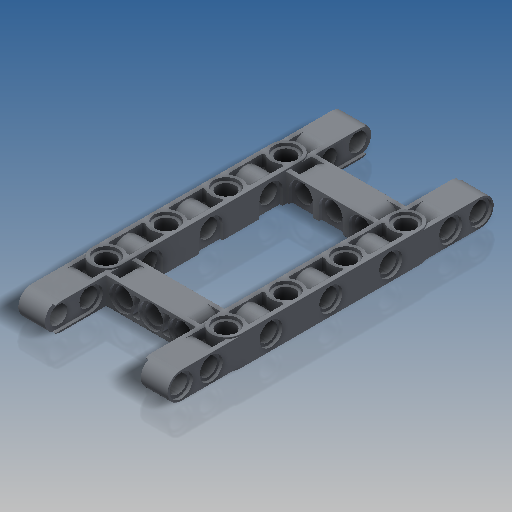
# Autodesk Inventor part: 64178-LtBluishGray
Saved by Autodesk Inventor 2018.3 (Build 223284000, 284)
## iProperties
Created: 2012-03-21
Part Number: 64178-LtBluishGray
Document SubType Name: Modeling
Designer: D. Kohfeld
Density: 1.06 g/cm^3
Material: ABS Plastic
Mass: 7.50717 g
Surface Area: 111.293 cm^2
Volume: 7.08223 cm^3
Appearance: LtBluishGray
Author: D. Kohfeld
Autodesk Inventor part; units mm, degrees
ref_plane "XZ Plane" through (0, 0, 0) normal (0, 1, 0) x (-1, 0, 0)
ref_plane "XY Plane" through (0, 0, 0) normal (0, 0, 1) x (1, 0, 0)
sketch "Sketch1" plane through (0, 0, 0) normal (0, 0, 1) x (1, 0, 0)
  line L0 (4, -24) -> (4, 24)
  line L1 (-4, 24) -> (-4, -24)
  arc A0 (4, 24) -> (-4, 24) centre (0, 24) ccw
  arc A1 (-4, -24) -> (4, -24) centre (0, -24) ccw
  circle A2 centre (0, 24) radius 3.2
  circle A3 centre (0, 24) radius 2.4
  line L2 (2.8284, 21.1716) -> (2.8284, 10.8284)
  line L3 (-2.8284, 21.1716) -> (-2.8284, 10.8284)
  arc A4 (-2.8284, 21.1716) -> (2.8284, 21.1716) centre (0, 24) ccw
  arc A5 (2.8284, 10.8284) -> (-2.8284, 10.8284) centre (0, 8) ccw
  circle A6 centre (0, 8) radius 3.2
  circle A7 centre (0, 8) radius 2.4
  line L4 (2.8284, 5.1716) -> (2.8284, -5.1716)
  line L5 (-2.8284, 5.1716) -> (-2.8284, -5.1716)
  arc A8 (-2.8284, 5.1716) -> (2.8284, 5.1716) centre (0, 8) ccw
  arc A9 (2.8284, -5.1716) -> (-2.8284, -5.1716) centre (0, -8) ccw
  circle A10 centre (0, -8) radius 3.2
  circle A11 centre (0, -8) radius 2.4
  line L6 (2.8284, -10.8284) -> (2.8284, -21.1716)
  line L7 (-2.8284, -10.8284) -> (-2.8284, -21.1716)
  arc A12 (-2.8284, -10.8284) -> (2.8284, -10.8284) centre (0, -8) ccw
  arc A13 (2.8284, -21.1716) -> (-2.8284, -21.1716) centre (0, -24) ccw
  circle A14 centre (0, -24) radius 3.2
  circle A15 centre (0, -24) radius 2.4
  line L8 (-4, -24) -> (-4, -40)
  line L9 (-4, -40) -> (-2.8284, -40)
  line L10 (-2.8284, -40) -> (-2.8284, -26.8284)
  line L11 (4, -24) -> (4, -40)
  line L12 (4, -40) -> (2.8284, -40)
  line L13 (2.8284, -40) -> (2.8284, -26.8284)
  line L14 (-4, 24) -> (-4, 40)
  line L15 (-4, 40) -> (-2.8284, 40)
  line L16 (-2.8284, 40) -> (-2.8284, 26.8284)
  line L17 (4, 24) -> (4, 40)
  line L18 (4, 40) -> (2.8284, 40)
  line L19 (2.8284, 40) -> (2.8284, 26.8284)
  line L20 (-2.8284, -40) -> (2.8284, -40)
  line L21 (-2.8284, 40) -> (2.8284, 40)
  line L22 (-2.8284, 21.1716) -> (0, 24) construction
  point P0 (0, 0)
  point P1 (-4, 0)
  dimension "d32" = 8
  dimension "d49" = 6.4
  dimension "d50" = 4.8
  dimension "d64" = 16
  dimension "d105" = 16
  dimension "d116" = 45
  constraints: 46 end point, 20 point on circle, 16 centre point, 10 parallel, 9 coincident, 8 tangent, 6 vertical alignment, 5 perpendicular, 4 equal radius, 3 equal length, 3 horizontal alignment, 3 vertical, 2 concentric, 1 midpoint, 28 other
  measures "d32" diameter of A0
  measures "d49" diameter of A2
  measures "d50" diameter of A3
  measures "d64" distance of L3.start L5.start
  measures "d105" vertical distance of L11.end A1.centre
  measures "d116" angle of L1 L22
extrude "Extrusion1" add sketch "Sketch1" along normal mid plane 8 contours A1 L1 A0 L0 | A2 | L2 A5 L3 A4 | A6 | L4 A9 L5 A8 | A10 | L6 A13 L7 A12 | A14
extrude "Extrusion18" add sketch "Sketch1" along normal mid plane 7.2 contours L11 L12 L13 A1 | A0 L19 L18 L17 | L10 L9 L8 A1 | A0 L14 L15 L16
sketch "Sketch6" plane through (0, 0, 4) normal (0, 0, 1) x (1, 0, 0)
  circle A0 centre (0, 24) radius 2.4 projected
  circle A1 centre (0, 24) radius 3.2 projected
  line L0 (2.8284, 21.1716) -> (2.8284, 10.8284) projected
  arc A2 (-2.8284, 21.1716) -> (2.8284, 21.1716) centre (0, 24) ccw projected
  arc A3 (2.8284, 10.8284) -> (-2.8284, 10.8284) centre (0, 8) ccw projected
  line L1 (-2.8284, 21.1716) -> (-2.8284, 10.8284) projected
  circle A4 centre (0, 8) radius 3.2 projected
  circle A5 centre (0, 24) radius 3.1 projected
  circle A6 centre (0, 8) radius 3.1 projected
  line L2 (4, 24) -> (4, -24) projected
  line L3 (4, -24) -> (4, 24) projected
  arc A7 (-2.8284, 5.1716) -> (2.8284, 5.1716) centre (0, 8) ccw projected
  line L4 (2.8284, 5.1716) -> (2.8284, -5.1716) projected
  arc A8 (2.8284, -5.1716) -> (-2.8284, -5.1716) centre (0, -8) ccw projected
  line L5 (-2.8284, 5.1716) -> (-2.8284, -5.1716) projected
  circle A9 centre (0, -8) radius 3.2 projected
  line L6 (2.8284, -10.8284) -> (2.8284, -21.1716) projected
  arc A10 (-2.8284, -10.8284) -> (2.8284, -10.8284) centre (0, -8) ccw projected
  line L7 (-2.8284, -10.8284) -> (-2.8284, -21.1716) projected
  arc A11 (2.8284, -21.1716) -> (-2.8284, -21.1716) centre (0, -24) ccw projected
  circle A12 centre (0, -24) radius 3.2 projected
  line L8 (4, -40) -> (4, -24) projected
  line L9 (4, -24) -> (4, -40) projected
  line L10 (4, 40) -> (4, 24) projected
  line L11 (4, 24) -> (4, 40) projected
extrude "Extrusion7" cut sketch "Sketch6" against normal blind 0.8 contours A0 | A1 | A4 | A5 | A6 | A9 | A12
extrude "Extrusion8" cut sketch "Sketch6" against normal blind 3.1 contours L0 A3 L1 A2 | A7 L4 A8 L5 | L6 A11 L7 A10
mirror "Mirror1" about plane through (0, 0, 0) normal (0, 0, 1) of "Extrusion7", "Extrusion8"
extrude "Extrusion19" add sketch "Sketch1" against normal up to surface (1.8 mm away) from surface at 0.9 contours L13 L20 L10 A1 | A0 L16 L21 L19
sketch "Sketch7" plane through (0, 0, 0) normal (1, 0, 0) x (0, 1, 0)
  line L0 (-21.1716, 0.9) -> (-10.8284, 0.9) projected
  line L1 (-21.1716, -0.9) -> (-10.8284, -0.9) projected
  circle A0 centre (-16, 0) radius 3.6
  circle A1 centre (-16, 0) radius 2.4
  circle A2 centre (0, 0) radius 3.6
  circle A3 centre (0, 0) radius 2.4
  circle A4 centre (16, 0) radius 3.6
  circle A5 centre (16, 0) radius 2.4
  line L2 (-16, 0) -> (0, 0) construction
  line L3 (0, 0) -> (16, 0) construction
  line L4 (-40, -3.6) -> (-40, 3.6) construction
  line L5 (40, -3.6) -> (40, 3.6) construction
  arc A6 (-40, 3.6) -> (-40, -3.6) centre (-40, 0) ccw
  arc A7 (40, -3.6) -> (40, 3.6) centre (40, 0) ccw
  line L6 (-40, 3.6) -> (-32, 3.6)
  arc A8 (-32, -3.6) -> (-32, 3.6) centre (-32, 0) ccw
  line L7 (-32, -3.6) -> (-40, -3.6)
  line L8 (40, 3.6) -> (32, 3.6)
  arc A9 (32, 3.6) -> (32, -3.6) centre (32, 0) ccw
  line L9 (32, -3.6) -> (40, -3.6)
  line L10 (-40, 0) -> (-32, 0) construction
  line L11 (32, 0) -> (40, 0) construction
  circle A10 centre (-40, 0) radius 3.2
  circle A11 centre (-32, 0) radius 3.2
  circle A12 centre (-32, 0) radius 2.4
  circle A13 centre (-40, 0) radius 2.4
  circle A14 centre (32, 0) radius 3.2
  circle A15 centre (40, 0) radius 3.2
  circle A16 centre (40, 0) radius 2.4
  circle A17 centre (32, 0) radius 2.4
  point P0 (-16, 0.9)
  dimension "d69" = 7.2
  dimension "d70" = 4.8
  dimension "d108" = 8
  dimension "d109" = 6.4
  dimension "d110" = 4.8
  constraints: 18 centre point, 16 end point, 12 coincident, 10 equal radius, 8 point on circle, 8 tangent, 5 parallel, 4 collinear, 3 midpoint, 1 horizontal alignment, 1 perpendicular, 1 vertical alignment
  measures "d69" diameter of A0
  measures "d70" diameter of A1
  measures "d108" distance of L10.end L10.start
  measures "d109" diameter of A10
  measures "d110" diameter of A13
extrude "Extrusion9" add sketch "Sketch7" against normal up to surface (8 mm away) from surface at 4 contours A0 L0 A1 | L0 A1 L1 A0 | A0 L1 A1 L0 | L1 A1 A0 | A2 | A4 | L6 A8 L7 A6 | L9 A9 L8 A7 | A10 | A11 | A14 | A15
extrude "Extrusion10" cut sketch "Sketch7" along normal through all both and the other way through all contours A1 L0 | L0 A1 L1 | L1 A1 | A3 | A5 | A12 | A13 | A16 | A17
sketch "Sketch8" plane through (4, -24, 4) normal (1, 0, 0) x (0, 0, -1)
  circle A0 centre (4, 24) radius 2.4 projected
  circle A1 centre (4, 8) radius 2.4 projected
  circle A2 centre (4, 40) radius 2.4 projected
  circle A3 centre (4, 8) radius 3.1
  circle A4 centre (4, 24) radius 3.1
  circle A5 centre (4, 40) radius 3.1
  circle A6 centre (4, 56) radius 2.4 projected
  circle A7 centre (4, -8) radius 2.4 projected
  arc A8 (0.4, -16) -> (7.6, -16) centre (4, -16) ccw projected
  arc A9 (7.6, 64) -> (0.4, 64) centre (4, 64) ccw projected
  circle A10 centre (4, 56) radius 3.1
  circle A11 centre (4, 64) radius 3.1
  circle A12 centre (4, -8) radius 3.1
  circle A13 centre (4, -16) radius 3.1
  dimension "d75" = 6.2
  constraints: 7 centre point, 7 coincident, 6 equal radius
  measures "d75" diameter of A3
extrude "Extrusion11" cut sketch "Sketch8" against normal blind 0.8
mirror "Mirror2" about plane through (0, 0, 0) normal (1, 0, 0) of "Extrusion11"
sketch "Sketch18" plane through (-4, -24, -4) normal (-1, 0, 0) x (0, 0, 1)
  circle A0 centre (4, 40) radius 3.1 projected
  circle A1 centre (4, 8) radius 3.1 projected
  circle A2 centre (4, 24) radius 3.1 projected
  line L0 (0, 48) -> (0, 0) projected
  line L1 (4, 43.1) -> (0, 43.1)
  line L2 (4, 36.9) -> (0, 36.9)
  line L3 (4, 27.1) -> (0, 27.1)
  line L4 (4, 20.9) -> (0, 20.9)
  line L5 (4, 11.1) -> (0, 11.1)
  line L6 (4, 4.9) -> (0, 4.9)
  constraints: 12 end point, 6 perpendicular, 6 point on circle, 6 point on line, 6 tangent
extrude "Extrusion26" cut sketch "Sketch18" against normal up to surface (0.8 mm away) contours A0 L2 L0 L1 | A1 L6 L0 L5 | A2 L4 L0 L3
sketch "Sketch15" plane through (-4, -24, -4) normal (-1, 0, 0) x (0, 0, 1)
  circle A0 centre (4, -16) radius 3.1 projected
  circle A1 centre (4, 64) radius 3.1 projected
  circle A2 centre (4, 56) radius 3.1 projected
  circle A3 centre (4, -8) radius 3.1 projected
  line L0 (0.4, 48) -> (0.4, 64) projected
  line L1 (0.4, -16) -> (0.4, 0) projected
  arc A4 (0.4, -16) -> (7.6, -16) centre (4, -16) ccw projected
  line L2 (7.6, 0) -> (7.6, -16) projected
  line L3 (7.6, 64) -> (7.6, 48) projected
  arc A5 (7.6, 64) -> (0.4, 64) centre (4, 64) ccw projected
  line L4 (0.9, 56) -> (0.9, 65.8303)
  line L5 (7.1, 56) -> (7.1, 65.8303)
  line L6 (0.9, -8) -> (0.9, -17.8303)
  line L7 (7.1, -8) -> (7.1, -17.8303)
  arc A6 (7.1, -8) -> (0.9, -8) centre (4, -8) ccw
  arc A7 (0.9, 56) -> (7.1, 56) centre (4, 56) ccw
  constraints: 12 point on circle, 8 end point, 8 tangent, 4 parallel, 2 centre point
extrude "Extrusion20" cut sketch "Sketch15" against normal up to surface (0.8 mm away) contours L7 A4 L6 A0 | A0 L6 A3 L7 | L5 A2 L4 A1 | A1 L4 A5 L5
fillet "Fillet2" radius 0.4 23 edges at (-2.8284, 21.1716, 2.45) (-2.8284, 10.8284, 2.45) (2.8284, 10.8284, 2.45) (2.8284, 21.1716, 2.45) (2.8284, 10.8284, -2.45) (2.8284, 21.1716, -2.45) (-2.8284, 21.1716, -2.45) (-2.8284, 10.8284, -2.45) (-2.8284, -21.1716, 2.45) (-2.8284, -10.8284, 2.45) (2.8284, -10.8284, 2.45) (2.8284, -10.8284, -2.45) (2.8284, -21.1716, 2.45) (2.8284, -21.1716, -2.45) (-2.8284, -21.1716, -2.45) (-2.8284, -10.8284, -2.45) (2.8284, -5.1716, 2.45) (2.8284, -5.1716, -2.45) (-2.8284, -5.1716, 2.45) (-2.8284, -5.1716, -2.45) (-2.8284, 5.1716, 2.45) (2.8284, 5.1716, 2.45) (2.8284, 5.1716, -2.45)
fillet "Fillet2" radius 0.1 11 edges at (-4, 0, 4) (0, 28, 4) (4, 0, 4) (0, -28, 4) (0, 28, -4) (-4, 8, -4) (-4, -8, -4) (-4, -21.55, -4) (-4, 21.55, -4) (0, -28, -4) (4, 0, -4)
ref_plane "Work Plane1" through (-16, 0, 0) normal (1, 0, 0) x (0, 1, 0)
sketch "Sketch11" plane through (0, 0, 0) normal (0, 0, 1) x (1, 0, 0)
  circle A0 centre (0, -24) radius 2.4 projected
  circle A1 centre (0, 24) radius 2.4 projected
  line L0 (-4, 40) -> (-4, 24) projected
  line L1 (-4, -24) -> (-4, -40) projected
  line L2 (-16, 56) -> (-16, -56) projected
  line L3 (-4, -26.8284) -> (-28, -26.8284)
  line L4 (-28, -26.8284) -> (-28, -28)
  line L5 (-28, -28) -> (-4, -28)
  line L6 (-4, -28) -> (-4, -26.8284)
  line L7 (-4, -20) -> (-28, -20)
  line L8 (-28, -20) -> (-28, -21.1716)
  line L9 (-28, -21.1716) -> (-4, -21.1716)
  line L10 (-4, -21.1716) -> (-4, -20)
  line L11 (-4, 28) -> (-28, 28)
  line L12 (-28, 28) -> (-28, 26.8284)
  line L13 (-28, 26.8284) -> (-4, 26.8284)
  line L14 (-4, 26.8284) -> (-4, 28)
  line L15 (-4, 21.1716) -> (-28, 21.1716)
  line L16 (-28, 21.1716) -> (-28, 20)
  line L17 (-28, 20) -> (-4, 20)
  line L18 (-4, 20) -> (-4, 21.1716)
  line L19 (-28, 21.1716) -> (-28, 26.8284) construction
  line L20 (-28, -26.8284) -> (-28, -21.1716) construction
  line L21 (-2.8284, 26.8284) -> (-2.8284, 32) projected
  line L22 (-2.8284, 32) -> (-4, 32) construction
  point P0 (0, 0)
  point P1 (-16, -20)
  point P2 (-28, -24)
  point P3 (-28, 24)
  dimension "d115" = 8
  constraints: 38 end point, 9 parallel, 8 equal length, 5 perpendicular, 5 point on line, 4 horizontal, 4 midpoint, 2 horizontal alignment
  measures "d115" distance between parallel lines of L7 L5
extrude "Extrusion13" add sketch "Sketch11" against normal up to surface (7.2 mm away) from surface at 3.6 contours L1 L5 L2 L3 | L2 L5 L4 L3 | L7 L10 L9 L2 | L2 L9 L8 L7
sketch "Sketch16" plane through (-28, -28, -3.6) normal (0, -1, 0) x (1, 0, 0)
  line L0 (24, 0) -> (0, 0) construction
  line L1 (24, 7.2) -> (0, 7.2) construction
  line L2 (0, 0) -> (0, 7.2) construction
  circle A0 centre (12, 3.6) radius 3.2
  circle A1 centre (12, 3.6) radius 2.4
  circle A2 centre (4, 3.6) radius 3.2
  circle A3 centre (4, 3.6) radius 2.4
  circle A4 centre (20, 3.6) radius 3.2
  circle A5 centre (20, 3.6) radius 2.4
  line L3 (4, 3.6) -> (12, 3.6) construction
  line L4 (12, 3.6) -> (20, 3.6) construction
  line L5 (4, 7.2) -> (20, 7.2)
  arc A6 (20, 0) -> (20, 7.2) centre (20, 3.6) ccw
  line L6 (20, 0) -> (4, 0)
  arc A7 (4, 7.2) -> (4, 0) centre (4, 3.6) ccw
  line L7 (24, 7.2) -> (24, 0) projected
  line L8 (6.5456, 6.1456) -> (9.4544, 6.1456)
  line L9 (6.5456, 1.0544) -> (9.4544, 1.0544)
  line L10 (14.5456, 6.1456) -> (17.4544, 6.1456)
  line L11 (14.5456, 1.0544) -> (17.4544, 1.0544)
  arc A8 (6.5456, 1.0544) -> (6.5456, 6.1456) centre (4, 3.6) ccw
  arc A9 (9.4544, 6.1456) -> (9.4544, 1.0544) centre (12, 3.6) ccw
  arc A10 (14.5456, 1.0544) -> (14.5456, 6.1456) centre (12, 3.6) ccw
  arc A11 (17.4544, 6.1456) -> (17.4544, 1.0544) centre (20, 3.6) ccw
  line L12 (4, 3.6) -> (6.5456, 6.1456) construction
  point P0 (28, 3.6)
  point P1 (12, 7.2)
  point P2 (0, 3.6)
  dimension "d117" = 8
  dimension "d118" = 4.8
  dimension "d119" = 6.4
  dimension "d126" = 45
  constraints: 18 end point, 12 centre point, 12 point on circle, 8 equal length, 8 equal radius, 7 coincident, 4 point on line, 4 tangent, 2 concentric, 2 midpoint, 2 perpendicular, 1 horizontal alignment, 1 vertical alignment
  measures "d117" distance of L3.start L3.end
  measures "d118" diameter of A3
  measures "d119" diameter of A2
  measures "d126" angle of L12 L3
extrude "Extrusion21" add sketch "Sketch16" against normal up to surface (8 mm away) contours A0 | A1 | A2 | A3 | A4 | A5 | L5 A6 L6 A7 | L8 A9 L9 A8 | L10 A11 L11 A10
extrude "Extrusion22" cut sketch "Sketch16" against normal through all contours A1 | A3 | A5
extrude "Extrusion23" cut sketch "Sketch16" against normal blind 0.8 contours A0 | A2 | A4
extrude "Extrusion24" cut sketch "Sketch16" against normal blind 6.2 contours L8 A9 L9 A8 | L10 A11 L11 A10
sketch "Sketch17" plane through (-28, -20, 3.6) normal (0, 1, 0) x (1, 0, 0)
  circle A0 centre (4, 3.6) radius 2.4 projected
  circle A1 centre (12, 3.6) radius 2.4 projected
  circle A2 centre (20, 3.6) radius 2.4 projected
  line L0 (0, 7.2) -> (24, 7.2) projected
  line L1 (0, 7.2) -> (0, 0) projected
  line L2 (0.8, 7.2) -> (0.8, 3.6)
  arc A3 (0.8, 3.6) -> (7.2, 3.6) centre (4, 3.6) ccw
  line L3 (7.2, 3.6) -> (7.2, 7.2)
  line L4 (8.8, 7.2) -> (8.8, 3.6)
  arc A4 (8.8, 3.6) -> (15.2, 3.6) centre (12, 3.6) ccw
  line L5 (15.2, 3.6) -> (15.2, 7.2)
  line L6 (16.8, 7.2) -> (16.8, 3.6)
  arc A5 (16.8, 3.6) -> (23.2, 3.6) centre (20, 3.6) ccw
  line L7 (23.2, 3.6) -> (23.2, 7.2)
  point P0 (28, 3.6)
  dimension "d129" = 6.4
  constraints: 12 end point, 6 point on circle, 6 point on line, 6 tangent, 3 centre point, 3 concentric, 3 parallel, 3 perpendicular, 2 equal radius
  measures "d129" diameter of A3
extrude "Extrusion25" cut sketch "Sketch17" against normal blind 0.8
fillet "Fillet3" radius 0.4 8 edges at (-21.4544, -24.9, 2.5456) (-18.5456, -24.9, 2.5456) (-21.4544, -24.9, -2.5456) (-18.5456, -24.9, -2.5456) (-13.4544, -24.9, -2.5456) (-13.4544, -24.9, 2.5456) (-10.5456, -24.9, 2.5456) (-10.5456, -24.9, -2.5456)
mirror "Mirror5" about plane through (0, 0, 0) normal (0, 1, 0) of "Extrusion24", "Extrusion25", "Extrusion22", "Extrusion23", "Extrusion13", "Extrusion21", "Fillet3"
mirror "Mirror3" about plane through (-16, 0, 0) normal (1, 0, 0) of "Extrusion7", "Extrusion1", "Extrusion11", "Mirror2", "Extrusion10", "Extrusion9", "Extrusion8", "Mirror1", "Fillet2", "Extrusion20", "Extrusion19", "Extrusion18", "Extrusion26"
fillet "Fillet4" radius 0.1 50 edges at (-36, -43.6, 0) (-36, -32, -3.6) (-36, -32, 3.6) (-28, -40.9487, 3.4728) (-28, -34, 3.6) (-28.4, -41.8303, 3.1) (-28, -40.9487, -3.4728) (-28, -34, -3.6) (-28.4, -41.8303, -3.1) (-4, -34, 3.6) (-4, -40.9487, 3.4728) (-3.6, -41.8303, 3.1) (-16, -28, 3.6) (-16, -20, 3.6) (-16, -28, -3.6) (4, -32, 3.6) (4, -32, -3.6) (4, -43.6, 0) (4, 43.6, 0) (4, 32, -3.6) (4, 32, 3.6) (-4, 40.9487, 3.4728) (-4, 34, 3.6) (-28, 40.9487, 3.4728) (-28, 34, 3.6) (-16, 28, 3.6) (-16, 20, 3.6) (-36, 43.6, 0) (-36, 32, -3.6) (-36, 32, 3.6) (-4, -40.9487, -3.4728) (-4, -34, -3.6) (-3.6, -41.8303, -3.1) (-4, 40.9487, -3.4728) (-4, 34, -3.6) (-3.6, 41.8303, -3.1) (-3.6, 41.8303, 3.1) (-28, 40.9487, -3.4728) (-28, 34, -3.6) (-16, 28, -3.6) (-12, -20, -3.6) (-4.4, -20, -3.6) (-20, -20, -3.6) (-4.4, 20, -3.6) (-12, 20, -3.6) (-20, 20, -3.6) (-28.4, 41.8303, -3.1) (-27.6, -20, -3.6) (-27.6, 20, -3.6) (-28.4, 41.8303, 3.1)
body "Solid1"
